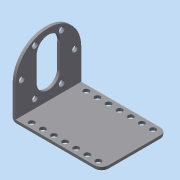
# Autodesk Inventor part: Motorhalterung
Saved by Autodesk Inventor 2014 SP2 (Build 180246200, 246)
## iProperties
Created: 2015-10-03
Part Number: Motorhalterung
Material: Generisch
Document SubType Name: Modeling
Designer: Home
Density: 1 g/cm^3
Appearance: Vorgabe
Author: Home
Autodesk Inventor part; units mm, degrees
ref_plane "YZ Plane" through (0, 0, 0) normal (1, 0, 0) x (0, 1, 0)
ref_plane "XZ Plane" through (0, 0, 0) normal (0, 1, 0) x (-1, 0, 0)
ref_plane "XY Plane" through (0, 0, 0) normal (0, 0, 1) x (1, 0, 0)
sketch "Skizze1" plane through (0, 0, 0) normal (0, 0, 1) x (1, 0, 0)
  line L0 (0, 0) -> (50.8, 0)
  line L1 (50.8, 0) -> (50.8, 37.59)
  line L2 (50.8, 37.59) -> (0, 37.59)
  line L3 (0, 37.59) -> (0, 0)
  dimension "d0" = 37.59
  dimension "d1" = 50.8
  constraints: 8 end point, 2 parallel, 1 horizontal, 1 perpendicular
  measures "d0" distance of L0.end L1.end
  measures "d1" distance of L1.end L2.end
extrude "Extrusion1" add sketch "Skizze1" along normal blind 1.59
sketch "Skizze4" plane through (0, 0, 0) normal (-1, 0, 0) x (0, 0, 1)
  line L0 (0, 37.59) -> (0, 0) projected
  line L1 (0, 0) -> (1.59, 0) projected
  line L2 (1.59, 37.59) -> (1.59, 0) projected
  line L3 (0, 37.59) -> (1.59, 37.59) projected
  line L4 (0, 37.59) -> (37.59, 37.59)
  line L5 (37.59, 37.59) -> (37.59, 0)
  line L6 (37.59, 0) -> (0, 0)
  line L7 (0, 0) -> (0, 37.59)
  dimension "d19" = 37.59
  constraints: 8 end point, 2 parallel, 1 horizontal, 1 perpendicular
  measures "d19" distance of L5.end L6.end
extrude "Extrusion2" add sketch "Skizze4" against normal blind 1.59 contours L4 L5 L6 L2
sketch "Skizze2" plane through (0, 0, 0) normal (-1, 0, 0) x (0, 0, 1)
  line L0 (0, 0) -> (1.59, 0) projected
  line L1 (1.59, 37.59) -> (1.59, 0) projected
  line L2 (0, 37.59) -> (18.59, 37.59)
  line L3 (37.59, 18.59) -> (37.59, 19)
  line L4 (18.59, 0) -> (0, 0)
  line L5 (0, 0) -> (0, 37.59)
  line L6 (37.59, 18.795) -> (-20.6317, 18.795) construction
  line L7 (26.59, 25.4) -> (12.57, 25.4)
  line L8 (12.57, 12.19) -> (26.59, 12.19)
  arc A0 (26.59, 12.19) -> (26.59, 25.4) centre (27.59, 18.795) ccw
  arc A1 (12.57, 25.4) -> (12.57, 12.19) centre (13.57, 18.795) ccw
  arc A2 (37.59, 18.59) -> (18.59, 37.59) centre (18.59, 18.59) ccw
  arc A3 (18.59, 0) -> (37.59, 19) centre (18.59, 19) ccw
  circle A4 centre (19.58, 18.795) radius 15.25 construction
  line L9 (19.58, 18.795) -> (19.58, 46.2315) construction
  circle A5 centre (32.7869, 26.42) radius 1.625
  circle A6 centre (32.7869, 11.17) radius 1.625
  circle A7 centre (19.58, 3.545) radius 1.625
  circle A8 centre (6.3731, 11.17) radius 1.625
  circle A9 centre (6.3731, 26.42) radius 1.625
  circle A10 centre (19.58, 34.045) radius 1.625
  line L10 (1.59, 0) -> (1.59, 37.59)
  point P0 (37.59, 37.59)
  point P1 (32.7869, 11.17)
  dimension "d4" = 37.59
  dimension "d5" = 14.02
  dimension "d6" = 13.21
  dimension "d8" = 11
  dimension "d9" = 19
  dimension "d10" = 30.5
  dimension "d13" = 360
  dimension "d15" = 3.25
  dimension "d16" = 3.25
  dimension "d17" = 3.25
  constraints: 18 end point, 11 centre point, 10 point on circle, 6 point on line, 5 coincident, 4 equal radius, 4 tangent, 3 parallel, 3 perpendicular, 2 collinear, 2 horizontal, 1 midpoint, 8 other
  measures "d4" distance of L2.start point (37.59, 37.59)
  measures "d5" distance of L7.start L7.end
  measures "d6" distance of L8.end L7.start
  measures "d8" distance from line of L3 L7.start
  measures "d9" radius of A2
  measures "d10" diameter of A4
  measures "d15" diameter of A5
  measures "d16" diameter of A6
  measures "d17" diameter of A7
extrude "Extrusion3" cut sketch "Skizze2" against normal blind 1.59 contours A0 L8 A1 L7 | A5 | A6 | A7 | A8 | A9 | A10
fillet "Rundung1" radius 18.5 2 edges at (0.795, 0, 37.59) (0.795, 37.59, 37.59)
fillet "Rundung2" radius 2 1 edges at (0, 18.795, 0)
fillet "Rundung3" radius 4 2 edges at (50.8, 0, 0.795) (50.8, 37.59, 0.795)
sketch "Skizze5" plane through (0, 0, 1.59) normal (0, 0, 1) x (1, 0, 0)
  line L0 (46.8, 37.59) -> (1.59, 37.59) projected
  line L1 (50.8, 4) -> (50.8, 33.59) projected
  line L2 (50.8, 18.795) -> (-11.9419, 18.795) construction
  point P0 (0, 0)
  point P1 (45.8, 34.415)
  point P2 (45.8, 3.175)
  dimension "d36" = 31.24
  dimension "d37" = 5
  dimension "d38" = 5
  dimension "d39" = 3.175
  constraints: 2 end point, 1 midpoint, 1 perpendicular
  measures "d36" distance of point (45.8, 3.175) point (45.8, 34.415)
  measures "d37" distance from line of L1 point (45.8, 34.415)
  measures "d38" distance from line of L1 point (45.8, 3.175)
  measures "d39" distance from line of L0 point (45.8, 34.415)
hole "Bohrung2" at (45.8, 34.415, 1.59) at (45.8, 3.175, 1.59) direction (0, 0, -1) diameter 3.25 end through all
pattern_linear "Rechteckige Anordnung1" count 7 spacing 6.35 along (-1, 0, 0) of "Bohrung2"
